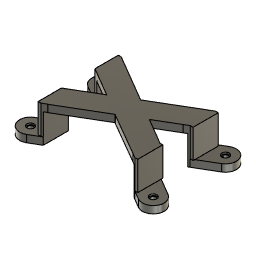
z_back_support (Autodesk Fusion 360 design; units mm, degrees)
Autodesk Fusion 360 part; units mm, degrees
note: some values were not read from the file. Chosen so that the rebuilt part matches the saved one: which bodies a step acts on; which face or edge a step refers to.
sketch "Sketch1" plane through (0, 0, 0) normal (0, 0, 1) x (1, 0, 0)
  line L0 (0, 0) -> (85, 0)
  line L1 (85, 0) -> (85, 50)
  line L2 (85, 50) -> (0, 50)
  line L3 (0, 50) -> (0, 0)
  line L4 (3.802651, -6.464507) -> (88.802651, 43.535493)
  arc A0 (88.802651, 43.535493) -> (81.197349, 56.464507) centre (85, 50) ccw
  line L5 (81.197349, 56.464507) -> (-3.802651, 6.464507)
  arc A1 (-3.802651, 6.464507) -> (3.802651, -6.464507) centre (0, 0) ccw
  line L6 (0, 0) -> (85, 50) construction
  line L7 (-3.802651, 43.535493) -> (81.197349, -6.464507)
  arc A2 (81.197349, -6.464507) -> (88.802651, 6.464507) centre (85, 0) ccw
  line L8 (88.802651, 6.464507) -> (3.802651, 56.464507)
  arc A3 (3.802651, 56.464507) -> (-3.802651, 43.535493) centre (0, 50) ccw
  line L9 (0, 50) -> (85, 0) construction
  dimension "d1" = 85
  dimension "d2" = 50
  dimension "d3" = 15
  dimension "d4" = 15
  constraint horizontal L0
  constraint vertical L1
  constraint horizontal L2
  constraint vertical L3
  constraint coincident L0.start L3.end
  constraint tangent L4 A0
  constraint tangent A0 L5
  constraint parallel L4 L5
  constraint tangent L5 A1
  constraint tangent L4 A1
  constraint coincident L1.end L2.start
  constraint tangent L7 A2
  constraint tangent A2 L8
  constraint parallel L7 L8
  constraint tangent L8 A3
  constraint tangent L7 A3
  constraint coincident L0.end L1.start
  constraint coincident L2.end L3.start
  measures "d1" distance of L0.start L0.end
  measures "d2" distance of L0.start L2.end
  measures "d3" diameter of A0
  measures "d4" diameter of A2
extrude "Extrude1" add sketch "Sketch1" along normal blind 5 contours L0 L3 L4 L5 L7 | L0 L3 L4 L5 A1 | L0 L1 L4 L7 L8 | L0 L1 L7 A2 L8 | L4 L5 L7 L8 | L2 L3 L7 L8 A3 | L2 L3 L5 L7 L8 | L1 L2 L4 L5 L8 | L1 L2 L4 A0 L5 picked at (28.333333, 13.766213) picked at (6.198321, -2.154836) picked at (56.666667, 13.766213) picked at (78.801679, -2.154836) picked at (37.569229, 25) picked at (6.198321, 52.154836) picked at (14.166667, 38.766213) picked at (56.666667, 36.233787) picked at (78.801679, 52.154836) makes body 1
sketch "Sketch2" plane through (0, 0, 5) normal (0, 0, 1) x (-1, 0, 0)
  arc A0 (-3.802651, -56.464507) -> (3.802651, -43.535493) centre (0, -50) ccw
  line L0 (3.802651, -43.535493) -> (-27.707688, -25)
  line L1 (-27.707688, -25) -> (3.802651, -6.464507)
  arc A1 (3.802651, -6.464507) -> (-3.802651, 6.464507) centre (0, 0) ccw
  line L2 (-3.802651, 6.464507) -> (-42.5, -16.29864)
  line L3 (-42.5, -16.29864) -> (-81.197349, 6.464507)
  arc A2 (-81.197349, 6.464507) -> (-88.802651, -6.464507) centre (-85, 0) ccw
  line L4 (-88.802651, -6.464507) -> (-57.292312, -25)
  line L5 (-57.292312, -25) -> (-88.802651, -43.535493)
  arc A3 (-88.802651, -43.535493) -> (-81.197349, -56.464507) centre (-85, -50) ccw
  line L6 (-81.197349, -56.464507) -> (-42.5, -33.70136)
  line L7 (-42.5, -33.70136) -> (-3.802651, -56.464507)
  point P0 (-85, -50)
  point P1 (-85, 0)
  point P2 (0, -50)
  constraint coincident A1.centre origin
  constraint coincident P0 A3.centre
  constraint coincident P1 A2.centre
  constraint coincident P2 A0.centre
hole "Hole1" at (0, 50, 5) at (0, 0, 5) at (85, 0, 5) at (85, 50, 5) direction (0, 0, -1) diameter 3.2 depth 300 tip angle 118 bodies 1
sketch "Sketch3" plane through (0, 0, 5) normal (0, 0, 1) x (-1, 0, 0)
  circle A0 centre (-85, 0) radius 1.6
  circle A1 centre (0, -50) radius 1.6
  circle A2 centre (0, 0) radius 1.6
  circle A3 centre (-85, -50) radius 1.6
  arc A4 (-3.802651, -56.464507) -> (3.802651, -43.535493) centre (0, -50) ccw
  line L0 (3.802651, -43.535493) -> (-27.707688, -25)
  line L1 (-27.707688, -25) -> (3.802651, -6.464507)
  arc A5 (3.802651, -6.464507) -> (-3.802651, 6.464507) centre (0, 0) ccw
  line L2 (-3.802651, 6.464507) -> (-42.5, -16.29864)
  line L3 (-42.5, -16.29864) -> (-81.197349, 6.464507)
  arc A6 (-81.197349, 6.464507) -> (-88.802651, -6.464507) centre (-85, 0) ccw
  line L4 (-88.802651, -6.464507) -> (-57.292312, -25)
  line L5 (-57.292312, -25) -> (-88.802651, -43.535493)
  arc A7 (-88.802651, -43.535493) -> (-81.197349, -56.464507) centre (-85, -50) ccw
  line L6 (-81.197349, -56.464507) -> (-42.5, -33.70136)
  line L7 (-42.5, -33.70136) -> (-3.802651, -56.464507)
  line L8 (-10, -69.730862) -> (-13, -69.730862)
  line L9 (-13, -69.730862) -> (-13, 37.485425)
  line L10 (-13, 37.485425) -> (-10, 37.485425)
  line L11 (-10, 37.485425) -> (-10, -69.730862)
  line L12 (-72, -69.419186) -> (-75, -69.419186)
  line L13 (-75, -69.419186) -> (-75, 44.342281)
  line L14 (-75, 44.342281) -> (-72, 44.342281)
  line L15 (-72, 44.342281) -> (-72, -69.419186)
  dimension "d10" = 3
  dimension "d11" = 3
  dimension "d12" = 10
  dimension "d13" = 10
  constraint horizontal L8
  constraint vertical L9
  constraint horizontal L10
  constraint vertical L11
  constraint horizontal L12
  constraint vertical L13
  constraint horizontal L14
  constraint vertical L15
  measures "d12" distance of A1.centre L11
  measures "d13" distance of A3.centre L13
extrude "Extrude2" cut sketch "Sketch3" against normal blind 313.82 contours L0 L7 L9 L11 | L1 L2 L9 L11 | L5 L6 L13 L15 | L3 L4 L13 L15 picked at (-12, -40.040723) picked at (-12, -9.959277) picked at (-74, -46.429865) picked at (-73, -9.959277) bodies 1 makes body 2 at (77.916357, 4.254097, 5) makes body 3 at (7.083643, 4.254097, 0) makes body 4 at (77.916357, 45.745903, 5) makes body 5 at (7.083643, 45.745903, 5)
move_body "Move1" bodies 1 to x (1, 0, 0) y (0, 1, 0) z (0, 0, 1) at (0, 0, 20)
extrude "Extrude3" add 1 faces at (10, 2.9819, 1.666667) along direction (1, 0, 0) blind 3 on bodies 3 bodies 3
extrude "Extrude4" add 1 faces at (10, 41.217194, 1.666667) along direction (1, 0, 0) blind 3 on bodies 5 bodies 5
extrude "Extrude5" add 2 faces at (75, 2.9819, 3.333333) (75, 47.0181, 1.666667) along direction (-1, 0, 0) blind 3 on bodies 2 4 bodies 2 4
sketch "Sketch4" plane through (0, 35.416287, 0) normal (0, -1, 0) x (1, 0, 0)
  line L0 (10, 5) -> (10, 0)
  line L1 (10, 0) -> (13, 0)
  line L2 (13, 0) -> (13, 5)
  line L3 (13, 5) -> (10, 5)
sketch "Sketch5" plane through (0, 0, 5) normal (0, 0, 1) x (-1, 0, 0)
  circle A0 centre (0, 0) radius 1.6
  line L0 (-10, -14.583713) -> (3.802651, -6.464507)
  arc A1 (3.802651, -6.464507) -> (-3.802651, 6.464507) centre (0, 0) ccw
  line L1 (-3.802651, 6.464507) -> (-10, 2.819007)
  line L2 (-10, 2.819007) -> (-13, 2.819007)
  line L3 (-13, 2.819007) -> (-13, -14.583713)
  line L4 (-13, -14.583713) -> (-10, -14.583713)
  line L5 (-10, -14.583713) -> (-13.418531, -16.594614)
  line L6 (-13.418531, -16.594614) -> (-13, -14.583713)
  line L7 (-10, 2.819007) -> (-13, 1.054301)
  line L8 (-13, 2.819007) -> (-10, 2.819007)
  line L9 (-13, 1.054301) -> (-13, 2.819007)
  constraint parallel L0 L5
  constraint parallel L1 L7
extrude "Extrude6" cut sketch "Sketch5" against normal blind 14.861 contours L2 L3 L7 L8 L9 picked at (-12, 2.230772) bodies 3
sketch "Sketch6" plane through (0, 0, 5) normal (0, 0, 1) x (-1, 0, 0)
  circle A0 centre (0, -50) radius 1.6
  line L0 (-10, -52.819007) -> (-3.802651, -56.464507)
  arc A1 (-3.802651, -56.464507) -> (3.802651, -43.535493) centre (0, -50) ccw
  line L1 (3.802651, -43.535493) -> (-10, -35.416287)
  line L2 (-10, -35.416287) -> (-13, -35.416287)
  line L3 (-13, -35.416287) -> (-13, -52.819007)
  line L4 (-13, -52.819007) -> (-10, -52.819007)
  line L5 (-10, -52.819007) -> (-13.8359, -50.562595)
  line L6 (-13.8359, -50.562595) -> (-13, -52.819007)
  line L7 (-75.074896, -52.822094) -> (-71.913856, -50.996056)
  line L8 (-71.913856, -50.996056) -> (-71.913856, -52.822094)
  line L9 (-71.913856, -52.822094) -> (-75.074896, -52.822094)
  line L10 (-75.074896, 2.879892) -> (-71.913856, 1.017274)
  line L11 (-71.913856, 1.017274) -> (-71.729073, 3.543956)
  line L12 (-71.729073, 3.543956) -> (-75.074896, 2.879892)
  constraint parallel L0 L5
  constraint vertical L8
  constraint perpendicular L8 L9
extrude "Extrude7" cut sketch "Sketch6" against normal blind 12.805 contours L3 L4 L5 | L7 L8 L9 | L10 L11 L12 picked at (-12, -52.230772) picked at (-72.967536, -52.213414) picked at (-72.905942, 2.480374) bodies 2 4 5
sketch "Sketch7" plane through (0, 0, 0) normal (0, 0, -1) x (1, 0, 0)
  line L0 (72, -51.045819) -> (75.074896, -52.822094)
  line L1 (75.074896, -52.822094) -> (75.005247, -52.822094)
  line L2 (75.005247, -52.822094) -> (81.197349, -56.464507)
  arc A0 (81.197349, -56.464507) -> (88.802651, -43.535493) centre (85, -50) ccw
  line L3 (88.802651, -43.535493) -> (75, -35.416287)
  line L4 (75, -35.416287) -> (72, -35.416287)
  line L5 (72, -35.416287) -> (72, -51.045819)
  circle A1 centre (85, -50) radius 1.6
  line L6 (13.027993, 0.444851) -> (13.027993, -16.35941)
  line L7 (13.027993, -16.35941) -> (10.003781, -14.579221)
  line L8 (10.003781, -14.579221) -> (10.003781, 2.703187)
  line L9 (10.003781, 2.703187) -> (13.027993, 0.922999)
  line L10 (13.027993, 0.922999) -> (13.027993, 0.444851)
  line L11 (71.987386, -16.332543) -> (75.132111, -14.476713)
  line L12 (75.132111, -14.476713) -> (75.132111, 2.878809)
  line L13 (75.132111, 2.878809) -> (72.00227, 1.065229)
  line L14 (72.00227, 1.065229) -> (71.987386, -16.332543)
  constraint vertical L6
  constraint parallel L6 L8
  constraint parallel L7 L9
  constraint parallel L6 L10
  constraint parallel L8 L12
extrude "Extrude8" add sketch "Sketch7" against normal up to surface (25 mm away) contours L6 L7 L8 L9 L10 | L11 L12 L13 L14 picked at (11.011851, -3.810394) picked at (73.040589, -9.914676) bodies 1 2 3
extrude "Extrude9" add sketch "Sketch4" along normal up to surface contours L0 L1 L2 L3 picked at (11, 3.333333) end surface through (75.132111, -2.878809, 0) normal (-0.50136073, -0.86523836, 0) offset 0 bodies 5
extrude "Extrude10" add 1 faces at (52.333333, 10.514326, 21.666667) along direction (-0.50702013, -0.86193422, 0) up to surface end surface through (75.132111, -2.878809, 0) normal (-0.50136073, -0.86523836, 0) offset 0 on bodies 1 bodies 1
sketch "Sketch8" plane through (0, 0, 0) normal (0, 0, -1) x (1, 0, 0)
  line L0 (3.802651, -56.464507) -> (13, -51.054301)
  line L1 (13, -51.054301) -> (13, -33.123525)
  line L2 (13, -33.123525) -> (10, -34.86187)
  line L3 (10, -34.86187) -> (10, -35.416287)
  line L4 (10, -35.416287) -> (-3.802651, -43.535493)
  arc A0 (-3.802651, -43.535493) -> (3.802651, -56.464507) centre (0, -50) ccw
  circle A1 centre (0, -50) radius 1.6
  line L5 (10, -35.416287) -> (13, -33.651581)
  line L6 (13, -30.881035) -> (8.967691, -33.252982)
  line L7 (8.967691, -33.252982) -> (10, -35.416287)
  constraint parallel L4 L5
  constraint parallel L5 L6
extrude "Extrude11" cut sketch "Sketch8" against normal blind 10.239 contours L1 L2 L3 L5 picked at (11, -34.643246) bodies 5
sketch "Sketch9" plane through (0, 0, 0) normal (0, 0, -1) x (1, 0, 0)
  circle A0 centre (0, -50) radius 1.6
  line L0 (13, -33.651581) -> (-3.802651, -43.535493)
  arc A1 (-3.802651, -43.535493) -> (3.802651, -56.464507) centre (0, -50) ccw
  line L1 (3.802651, -56.464507) -> (13, -51.054301)
  line L2 (13, -51.054301) -> (13, -33.651581)
  line L3 (13, -33.651581) -> (9.109894, -35.939879)
  line L4 (9.109894, -53.342599) -> (13, -51.054301)
  line L5 (10, -35.416287) -> (10, -52.819007)
  line L6 (71.888367, -33.598997) -> (75.100607, -35.491479)
  line L7 (75.100607, -35.491479) -> (75.100607, -52.862752)
  line L8 (75.100607, -52.862752) -> (71.987701, -51.028792)
  line L9 (71.987701, -51.028792) -> (71.987701, -33.65752)
  dimension "d35" = 3
  dimension "d36" = 3.112905
  constraint parallel L0 L3
  constraint parallel L1 L4
  constraint parallel L2 L5
  constraint vertical L7
  constraint parallel L6 L8
  constraint parallel L7 L9
  measures "d35" distance of L2 L5
  measures "d36" distance of L7 L9
extrude "Extrude12" add sketch "Sketch9" against normal up to surface (25 mm away) contours L0 L1 L2 L3 L4 L5 | L6 L7 L8 L9 picked at (11, -46.429865) picked at (73.025336, -40.059264) bodies 1 4 5
sketch "Sketch10" plane through (0, 0, 5) normal (0, 0, 1) x (-1, 0, 0)
  circle A0 centre (0, -50) radius 1.6
  line L0 (-10, -35.416287) -> (-10, -52.819007)
  line L1 (-10, -52.819007) -> (-3.802651, -56.464507)
  arc A1 (-3.802651, -56.464507) -> (3.802651, -43.535493) centre (0, -50) ccw
  line L2 (3.802651, -43.535493) -> (-10, -35.416287)
  point P0 (0, -50)
  constraint coincident P0 A0.centre
hole "Hole2" at (0, 50, 5) at (0, 0, 5) direction (0, 0, -1) diameter 3.4 depth 15 tip angle 118 bodies 1
sketch "Sketch11" plane through (0, 0, 5) normal (0, 0, 1) x (-1, 0, 0)
  line L0 (-75.100607, -35.491479) -> (-74.972977, -35.416287)
  line L1 (-74.972977, -35.416287) -> (-75, -35.416287)
  line L2 (-75, -35.416287) -> (-88.802651, -43.535493)
  arc A0 (-88.802651, -43.535493) -> (-81.197349, -56.464507) centre (-85, -50) ccw
  line L3 (-81.197349, -56.464507) -> (-75.005247, -52.822094)
  line L4 (-75.005247, -52.822094) -> (-75.031594, -52.822094)
  line L5 (-75.031594, -52.822094) -> (-75.100607, -52.862752)
  line L6 (-75.100607, -52.862752) -> (-75.100607, -35.491479)
  circle A1 centre (-85, -50) radius 1.6
  circle A2 centre (-85, 0) radius 1.6
  point P0 (-85, -50)
  point P1 (-85, -0.0001)
  dimension "d42" = 0.0001
  constraint coincident P0 A0.centre
  measures "d42" distance of P1 A2.centre
hole "Hole3" at (85, 50, 5) at (85, 0.0001, 5) direction (0, 0, -1) diameter 3.4 depth 15 tip angle 118 bodies 1
extrude "Extrude13" add 1 faces at (75.100607, 41.281904, 11.666667) along direction (1, 0, 0) blind 2 on bodies 1 bodies 1
extrude "Extrude14" add 1 faces at (75.132111, 8.691539, 11.666667) along direction (1, 0, 0) blind 2 on bodies 1 bodies 1
extrude "Extrude15" add 1 faces at (10.003781, 8.818419, 11.666667) along direction (-1, 0, 0) blind 2 on bodies 1 bodies 1
extrude "Extrude16" add 1 faces at (10, 41.217194, 11.666667) along direction (-1, 0, 0) blind 2 on bodies 1 bodies 1
extrude "Extrude17" cut 1 faces at (13.027993, 4.837804, 6.666667) along direction (-1, 0, 0) blind 2 on bodies 1 bodies 1
extrude "Extrude18" cut 1 faces at (13, 45.253395, 6.666667) along direction (-1, 0, 0) blind 2 on bodies 1 bodies 1
extrude "Extrude19" cut 1 faces at (71.991591, 11.417687, 8.333333) along direction (0.99999963, 0.00085548, 0) blind 2 on bodies 1 bodies 1
extrude "Extrude20" cut 1 faces at (71.987701, 45.238368, 6.666667) along direction (1, 0, 0) blind 2 on bodies 1 bodies 1
extrude "Extrude21" cut 1 faces at (72.666666, 1.588545, 1.666667) along direction (0.00085548, -0.99999963, 0) blind 77.235 on bodies 1 bodies 1
extrude "Extrude22" cut 1 faces at (72.668936, -1.064658, 11.666667) along direction (0.00085548, -0.99999963, 0) blind 27.518 on bodies 1 bodies 1 makes body 6 at (72.001514, -0.182209, 1.666667)
extrude "Extrude23" cut 1 faces at (72, -0.182697, 3.333333) along direction (1, 0, 0) blind 0.737 on bodies 6 bodies 6
extrude "Extrude24" cut 1 faces at (72.000757, -1.068033, 3.333333) along direction (0, -1, 0) blind 0.155 on bodies 6 bodies 6
extrude "Extrude25" cut 1 faces at (72.654368, 51.028792, 6.666667) along direction (0, 1, 0) blind 49.094 on bodies 1 bodies 1
extrude "Extrude26" cut 1 faces at (12.333333, 51.054301, 13.333333) along direction (0, 1, 0) blind 33.233 on bodies 1 bodies 1
extrude "Extrude27" cut 1 faces at (12.361326, -0.922999, 6.666667) along direction (0, -1, 0) blind 74.709 on bodies 1 bodies 1
extrude "Extrude28" cut 1 faces at (8.666667, 35.808444, 5) along direction (0, 0, 1) blind 30.306 on bodies 1 bodies 1
extrude "Extrude29" cut 1 faces at (8.666642, 14.189303, 5) along direction (0, 0, 1) blind 31.02 on bodies 1 bodies 1
extrude "Extrude30" add 1 faces at (72, 0.707216, 23.333333) along direction (1, 0, 0) blind 2.728 on bodies 1 bodies 1 6
extrude "Extrude31" add 1 faces at (73.333333, 1.589116, 23.333333) along direction (0.00085548, -0.99999963, 0) blind 0.007 on bodies 1 bodies 1
extrude "Extrude32" add 1 faces at (72.66742, -1.054301, 23.333333) along direction (0, -1, 0) up to surface (1.824508 mm away) on bodies 1 bodies 1
extrude "Extrude33" add 1 faces at (74.002261, -1.662471, 23.333333) along direction (1, 0, 0) blind 1.492 on bodies 1 bodies 1
sketch "Sketch12" plane through (0, 0, 25) normal (0, 0, 1) x (-1, 0, 0)
  line L0 (-72, 2.878809) -> (-77.132111, 2.878809)
  line L1 (-77.132111, 2.878809) -> (-77.132111, -14.476713)
  line L2 (-77.132111, -14.476713) -> (-75.132111, -14.476713)
  line L3 (-75.132111, -14.476713) -> (-72, -16.325099)
  line L4 (-72, -16.325099) -> (-72, -16.348419)
  line L5 (-72, -16.348419) -> (-57.292312, -25)
  line L6 (-57.292312, -25) -> (-72, -33.651581)
  line L7 (-72, -33.651581) -> (-72, -33.664765)
  line L8 (-72, -33.664765) -> (-75.100607, -35.491479)
  line L9 (-75.100607, -35.491479) -> (-77.100607, -35.491479)
  line L10 (-77.100607, -35.491479) -> (-77.100607, -52.862752)
  line L11 (-77.100607, -52.862752) -> (-75.100607, -52.862752)
  line L12 (-75.100607, -52.862752) -> (-72, -51.036038)
  line L13 (-72, -51.036038) -> (-72, -51.054301)
  line L14 (-72, -51.054301) -> (-42.5, -33.70136)
  line L15 (-42.5, -33.70136) -> (-10, -52.819007)
  line L16 (-10, -52.819007) -> (-8, -52.819007)
  line L17 (-8, -52.819007) -> (-8, -36.592758)
  line L18 (-8, -36.592758) -> (-27.707688, -25)
  line L19 (-27.707688, -25) -> (-13, -16.348419)
  line L20 (-13, -16.348419) -> (-13, -16.342932)
  line L21 (-13, -16.342932) -> (-10.003781, -14.579221)
  line L22 (-10.003781, -14.579221) -> (-9.992364, -14.579221)
  line L23 (-9.992364, -14.579221) -> (-8.003781, -13.409466)
  line L24 (-8.003781, -13.409466) -> (-8.003781, 2.703187)
  line L25 (-8.003781, 2.703187) -> (-10.003781, 2.703187)
  line L26 (-10.003781, 2.703187) -> (-13, 0.939476)
  line L27 (-13, 0.939476) -> (-13, 1.054301)
  line L28 (-13, 1.054301) -> (-42.5, -16.29864)
  line L29 (-42.5, -16.29864) -> (-42.382062, -16.098145)
  line L30 (-42.382062, -16.098145) -> (-71.995783, 1.06147)
  line L31 (-71.995783, 1.06147) -> (-72, 1.054301)
  line L32 (-72, 1.054301) -> (-72, 2.878809)
  line L33 (-72, 1.054301) -> (-75.864184, 3.327351)
  line L34 (-75.864184, 3.327351) -> (-73.367239, 4.606076)
  line L35 (-73.367239, 4.606076) -> (-69.698872, 3.546762)
  line L36 (-69.698872, 3.546762) -> (-72, 1.054301)
  constraint perpendicular L31 L33
extrude "Extrude34" cut sketch "Sketch12" against normal blind 7.866 contours L0 L32 L33 picked at (-73.033888, 2.27064) bodies 1
sketch "Sketch13" plane through (0, 0, 5) normal (0, 0, 1) x (-1, 0, 0)
  circle A0 centre (-85, -0.0001) radius 1.7
  line L0 (-74.003262, 2.2247) -> (-74.003283, 2.248452)
  line L1 (-74.003283, 2.248452) -> (-74.971568, 2.819007)
  line L2 (-74.971568, 2.819007) -> (-75, 2.819007)
  line L3 (-75, 2.819007) -> (-81.197349, 6.464507)
  arc A1 (-81.197349, 6.464507) -> (-88.802651, -6.464507) centre (-85, 0) ccw
  line L4 (-88.802651, -6.464507) -> (-77.132111, -13.32953)
  line L5 (-77.132111, -13.32953) -> (-77.132111, 2.878809)
  line L6 (-77.132111, 2.878809) -> (-75.132111, 2.878809)
  line L7 (-75.132111, 2.878809) -> (-74.003262, 2.2247)
  point P0 (-85, 0)
  point P1 (0, -50.029447)
  point P2 (-85, -50.029447)
  constraint coincident P0 A1.centre
hole "Hole4" at (0, 50.029447, 5) at (85, 50.029447, 5) at (0, 0, 5) at (85, 0, 5) direction (0, 0, -1) diameter 3.4 depth 11 tip angle 118 counterbore diameter 5 counterbore depth 1 bodies 1
